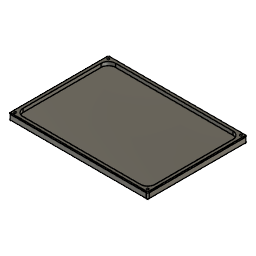
arm_holder_weight (アセンブリ) (Autodesk Fusion 360 archive; units mm, degrees)
design "arm_holder_weight_holder"
Autodesk Fusion 360 part; units mm, degrees
sketch "スケッチ1" plane through (0, 0, 0) normal (0, 0, 1) x (1, 0, 0)
  line L0 (91.25, 64) -> (-91.25, 64)
  line L1 (-91.25, 64) -> (-91.25, -64)
  line L2 (-91.25, -64) -> (91.25, -64)
  line L3 (91.25, -64) -> (91.25, 64)
  line L4 (91.25, 64) -> (-91.25, -64) construction
  line L5 (-91.25, 64) -> (91.25, -64) construction
  line L6 (96.25, -69) -> (-96.25, -69)
  line L7 (-96.25, -69) -> (-96.25, 69)
  line L8 (-96.25, 69) -> (96.25, 69)
  line L9 (96.25, 69) -> (96.25, -69)
  line L10 (96.25, -69) -> (-96.25, 69) construction
  line L11 (-96.25, -69) -> (96.25, 69) construction
  dimension "d1" = 182.5
  dimension "d2" = 128
  dimension "d3" = 192.5
  dimension "d4" = 138
  constraint horizontal L0
  constraint perpendicular L0 L1
  constraint parallel L0 L2
  constraint parallel L1 L3
  constraint coincident L4 origin
  constraint coincident L5 origin
  constraint horizontal L6
  constraint perpendicular L6 L7
  constraint parallel L6 L8
  constraint parallel L7 L9
  constraint coincident L10 origin
  constraint coincident L11 origin
  measures "d1" distance of L1.end L2.end
  measures "d2" distance of L0.end L1.end
  measures "d3" distance of L7.end L8.end
  measures "d4" distance of L6.end L7.end
extrude "押し出し1" add sketch "スケッチ1" along normal blind 5 contours L0 L1 L2 L3
extrude "押し出し2" add sketch "スケッチ1" along normal blind 10
fillet "フィレット2" radius 10 4 edges at (-91.25, 64, 7.5) (-91.25, -64, 7.5) (91.25, -64, 7.5) (91.25, 64, 7.5)
sketch "スケッチ2" plane through (0, 0, 10) normal (0, 0, 1) x (-1, 0, 0)
  line L0 (-96.25, -69) -> (96.25, -69)
  line L1 (96.25, -69) -> (96.25, 69)
  line L2 (96.25, 69) -> (-96.25, 69)
  line L3 (-96.25, 69) -> (-96.25, -69)
  line L4 (96.25, -69) -> (91.75, -69)
  line L5 (91.75, -69) -> (91.75, -64.5)
  line L6 (91.75, -64.5) -> (96.25, -64.5)
  line L7 (96.25, -64.5) -> (96.25, -69)
  line L8 (0, -2.5) -> (0, -20)
  line L9 (-91.75, -64.5) -> (-96.25, -64.5)
  line L10 (-91.75, -69) -> (-91.75, -64.5)
  line L11 (-20, 0) -> (-2.5, 0)
  line L12 (91.75, 64.5) -> (96.25, 64.5)
  line L13 (91.75, 69) -> (91.75, 64.5)
  line L14 (-91.75, 69) -> (-91.75, 64.5)
  line L15 (-91.75, 64.5) -> (-96.25, 64.5)
  line L16 (-91.25, -54) -> (-91.25, 54)
  line L17 (-81.25, 64) -> (81.25, 64)
  line L18 (91.25, 54) -> (91.25, -54)
  line L19 (81.25, -64) -> (-81.25, -64)
  arc A0 (-81.25, 64) -> (-91.25, 54) centre (-81.25, 54) ccw
  arc A1 (91.25, 54) -> (81.25, 64) centre (81.25, 54) ccw
  arc A2 (81.25, -64) -> (91.25, -54) centre (81.25, -54) ccw
  arc A3 (-91.25, -54) -> (-81.25, -64) centre (-81.25, -54) ccw
  dimension "d11" = 4.5
  dimension "d12" = 4.5
  constraint horizontal L4
  constraint vertical L5
  constraint horizontal L6
  constraint vertical L7
  constraint coincident L0.end L1.start
  constraint symmetric L4.end L8 L10.start
  constraint symmetric L5.end L8 L9.start
  constraint symmetric L6.end L8 L9.end
  constraint symmetric L4.end L11 L13.start
  constraint symmetric L5.end L11 L12.start
  constraint symmetric L6.end L11 L12.end
  constraint symmetric L9.start L11 L14.end
  constraint symmetric L9.end L11 L15.end
  constraint symmetric L10.start L11 L14.start
  measures "d11" distance of L0.end L4.end
  measures "d12" distance of L0.end L6.end
hole "穴1" at (-91.75, 64.5, 10) at (91.75, 64.5, 10) at (-91.75, -64.5, 10) at (91.75, -64.5, 10) direction (0, 0, -1) diameter 2.93 depth 4 tip angle 180
thread "ねじ1" "ISO Metric profile 3.5 M3.5x0.6 M3.5x0.6 6H" major diameter 3.5995 minor diameter 2.93 pitch 0.6 angle 60 resizes the face on face at (-93.2145, -64.5365, 8.6667) on face at (-93.2145, 64.4635, 8.6667) on face at (90.2855, 64.4635, 8.6667) on face at (90.2855, -64.5365, 8.6667)
fillet "フィレット3" radius 2 8 edges at (0, -69, 0) (-96.25, 0, 0) (0, 69, 0) (96.25, 0, 0) (96.25, -69, 5) (-96.25, -69, 5) (-96.25, 69, 5) (96.25, 69, 5)
fillet "フィレット3" radius 1 4 edges at (0, -69, 10) (-96.25, 0, 10) (0, 69, 10) (96.25, 0, 10)

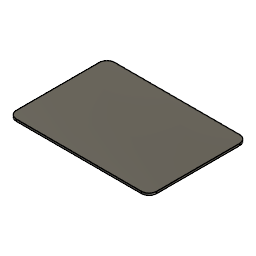
design "arm_holder_weight"
Autodesk Fusion 360 part; units mm, degrees
sketch "スケッチ1" plane through (0, 0, 0) normal (0, 0, 1) x (1, 0, 0)
  line L0 (-91, 63.75) -> (91, 63.75)
  line L1 (91, 63.75) -> (91, -63.75)
  line L2 (91, -63.75) -> (-91, -63.75)
  line L3 (-91, -63.75) -> (-91, 63.75)
  line L4 (-91, 63.75) -> (91, -63.75) construction
  line L5 (91, 63.75) -> (-91, -63.75) construction
  dimension "d1" = 182
  dimension "d2" = 127.5
  constraint horizontal L0
  constraint perpendicular L0 L1
  constraint parallel L0 L2
  constraint parallel L1 L3
  constraint coincident L4 origin
  constraint coincident L5 origin
  measures "d1" distance of L1.end L2.end
  measures "d2" distance of L0.end L1.end
extrude "押し出し1" add sketch "スケッチ1" along normal blind 2.5
fillet "フィレット1" radius 10 4 edges at (91, -63.75, 1.25) (91, 63.75, 1.25) (-91, 63.75, 1.25) (-91, -63.75, 1.25)
